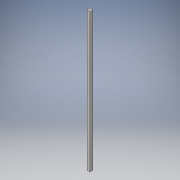
# Autodesk Inventor part: Glue-on .25in post to make up for our mistake
Saved by Autodesk Inventor 2016 (Build 200138000, 138)
## iProperties
Created: 2018-02-03
Part Number: Glue-on .25in post to make up for our mistake
Material: Generic
Document SubType Name: Modeling
Designer: dash
Density: 1 g/cm^3
Appearance: Default
Author: dash
Autodesk Inventor part; units mm, degrees
ref_plane "YZ Plane" through (0, 0, 0) normal (1, 0, 0) x (0, 1, 0)
ref_plane "XZ Plane" through (0, 0, 0) normal (0, 1, 0) x (-1, 0, 0)
ref_plane "XY Plane" through (0, 0, 0) normal (0, 0, 1) x (1, 0, 0)
sketch "Sketch1" plane through (0, 0, 0) normal (0, 0, 1) x (1, 0, 0)
  line L0 (-4.9659, 0.4493) -> (1.3841, 0.4493)
  line L1 (1.3841, 0.4493) -> (1.3841, -298.0007)
  line L2 (1.3841, -298.0007) -> (-4.9659, -298.0007)
  line L3 (-4.9659, -298.0007) -> (-4.9659, 0.4493)
  point P0 (0, 0)
  dimension "d0" = 6.35
  dimension "d1" = 298.45
  constraints: 8 end point, 2 parallel, 1 horizontal, 1 perpendicular
  measures "d0" distance of L1.end L2.end
  measures "d1" distance of L0.end L1.end
extrude "Extrusion1" add sketch "Sketch1" along normal blind 6.35
body "Solid1"
